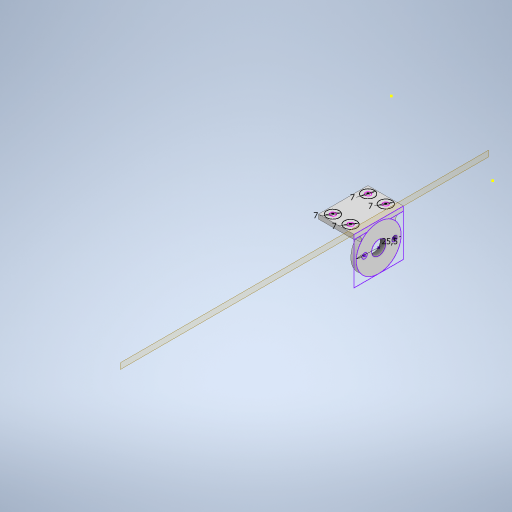
# Autodesk Inventor part: крепёж_мотора_прототип
Saved by Autodesk Inventor 2023 (Build 270158000, 158)
## iProperties
Created: 2025-12-12
Part Number: крепёж_мотора_прототип
Material: Типовые
Document SubType Name: Modeling
Designer: garin
Density: 1 g/cm^3
Appearance: По умолчанию
Author: garin
Autodesk Inventor part; units mm, degrees
ref_plane "YZ Plane" through (0, 0, 0) normal (1, 0, 0) x (0, 1, 0)
ref_plane "XZ Plane" through (0, 0, 0) normal (0, 1, 0) x (-1, 0, 0)
ref_plane "XY Plane" through (0, 0, 0) normal (0, 0, 1) x (1, 0, 0)
ref_plane "РабПлоскость1" through (57.3886, 15.9976, 24.7396) normal (1, 0, 0) x (0, 1, 0)
sketch "Эскиз1" plane through (57.3886, 15.9976, 24.7396) normal (1, 0, 0) x (0, 1, 0)
  circle A0 centre (-16.5, 48) radius 1.5
  circle A1 centre (-16.5, 31) radius 1.5
  circle A2 centre (-16.5, 40) radius 4
  line L0 (-3, 26) -> (-3, 54)
  circle A3 centre (-16.5, 40) radius 12.75
  line L1 (-3, 54) -> (-3, 26)
  line L2 (-3, 27.25) -> (-3, 52.75)
  line L3 (-3, 26) -> (-29.25, 26)
  line L4 (-29.25, 26) -> (-29.25, 54)
  line L5 (-29.25, 54) -> (-3, 54)
  line L6 (-3, 54) -> (-3, 26)
  line L7 (-5.5313, 46.5) -> (-5.5313, 54)
  line L8 (-3, 54) -> (-3, 26)
  line L9 (-5.5313, 26) -> (-5.5313, 33.5)
  point P0 (-15.9976, -24.7396)
  point P1 (-3, 26)
  dimension "d15" = 25.5
  constraints: 20 end point, 5 point on line, 4 centre point, 4 equal length, 2 point on circle, 1 coincident, 1 horizontal, 1 perpendicular, 1 vertical
  measures "d15" diameter of A3
extrude "Выдавливание1" add sketch "Эскиз1" against normal blind 3 contours A3
extrude "Выдавливание2" add sketch "Эскиз1" against normal blind 20 contours L3 L9 A3 L7 L5 L0
fillet "Сопряжение1" radius 2 1 edges at (55.8886, 10.4663, 58.2396)
fillet "Сопряжение2" radius 2 1 edges at (55.8886, 10.4663, 71.2396)
sketch "Эскиз2" plane through (57.3886, 12.9976, 78.7396) normal (0, 1, 0) x (1, 0, 0)
  point P0 (-57.3886, 78.7396)
sketch "Эскиз4" plane through (57.3886, 12.9976, 78.7396) normal (0, 1, 0) x (1, 0, 0)
  circle A0 centre (-6, 24) radius 1.5 projected
  circle A1 centre (-6, 24) radius 3.5
  circle A2 centre (-6, 4) radius 1.5 projected
  circle A3 centre (-6, 4) radius 3.5
  circle A4 centre (-16, 4) radius 1.5 projected
  circle A5 centre (-16, 4) radius 3.5
  circle A6 centre (-16, 24) radius 1.5 projected
  circle A7 centre (-16, 24) radius 3.5
  point P0 (-57.3886, 78.7396)
  dimension "d33" = 7
  dimension "d34" = 7
  dimension "d35" = 7
  dimension "d36" = 7
  constraints: 4 centre point, 4 coincident
  measures "d33" diameter of A1
  measures "d34" diameter of A3
  measures "d35" diameter of A5
  measures "d36" diameter of A7
extrude "Выдавливание5" cut sketch "Эскиз4" against normal blind 2 from surface at -2.5313
